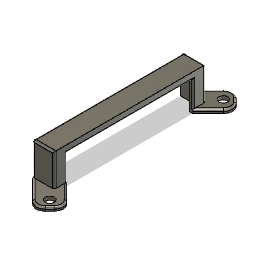
halterung_hdbaset_sender v1 (Autodesk Fusion 360 design; units mm, degrees)
Autodesk Fusion 360 part; units mm, degrees
note: some values were not read from the file. Chosen so that the rebuilt part matches the saved one: which pieces of a blend or face edit are solid.
sketch "Skizze1" plane through (0, 0, 0) normal (1, 0, 0) x (0, 0, -1)
  line L0 (0, 0) -> (0, 18)
  line L1 (0, 18) -> (80, 18)
  line L2 (80, 18) -> (80, 0)
  line L3 (0, 0) -> (-2, 0)
  line L4 (-2, 0) -> (-2, 20)
  line L5 (-2, 20) -> (82, 20)
  line L6 (82, 20) -> (82, 0)
  line L7 (82, 0) -> (80, 0)
  dimension "d1" = 18
  dimension "d2" = 80
  dimension "d3" = 18
  dimension "d4" = 2
  dimension "d5" = 20
  dimension "d6" = 84
  constraint coincident L0.start L3.start
  constraint vertical L0
  constraint perpendicular L0 L1
  constraint perpendicular L1 L2
  constraint perpendicular L0 L3
  constraint perpendicular L3 L4
  constraint perpendicular L4 L5
  constraint perpendicular L3 L6
  constraint perpendicular L2 L7
  measures "d1" distance of L0.start L0.end
  measures "d2" distance of L0.end L1.end
  measures "d3" distance of L1.end L2.end
  measures "d4" distance of L0.start L3.end
  measures "d5" distance of L3.end L4.end
  measures "d6" distance of L4.end L5.end
extrude "Extrusion1" add sketch "Skizze1" along normal blind 10
sketch "Skizze2" plane through (10, 0, 0) normal (1, 0, 0) x (0, 0, -1)
  line L0 (0, 0) -> (0, 18)
  line L1 (0, 18) -> (80, 18)
  line L2 (80, 18) -> (80, 0)
  line L3 (80, 0) -> (82, 0)
  line L4 (82, 0) -> (82, 20)
  line L5 (82, 20) -> (-2, 20)
  line L6 (-2, 20) -> (-2, 0)
  line L7 (-2, 0) -> (0, 0)
  line L8 (-2, 20) -> (-2, 0)
  line L9 (-2, 0) -> (5, 0)
  line L10 (5, 0) -> (5, 16)
  line L11 (5, 16) -> (75, 16)
  line L12 (75, 16) -> (75, 0)
  line L13 (75, 0) -> (82, 0)
  line L14 (82, 20) -> (82, 0)
  line L15 (82, 20) -> (-2, 20)
  dimension "d9" = 7
  dimension "d10" = 16
  dimension "d11" = 7
  constraint coincident L5.end L6.start
  constraint coincident L6.end L7.start
  constraint perpendicular L0 L9
  constraint perpendicular L9 L10
  constraint perpendicular L10 L11
  constraint perpendicular L1 L12
  constraint coincident L3.end L4.start
  constraint perpendicular L4 L13
  constraint coincident L4.end L5.start
  measures "d9" distance of L6.end L9.end
  measures "d10" distance of L9.end L10.end
  measures "d11" distance of L12.end L3.end
extrude "Extrusion2" add sketch "Skizze2" along normal blind 2
ref_plane "Arbeitsebene1" through (6, 0, -1.5) normal (0, -1, 0) x (0, 0, -1)
sketch "Skizze3" plane through (6, 0, -1.5) normal (0, -1, 0) x (1, 0, 0)
  line L0 (-6, 3.5) -> (4.949747, 14.449747)
  line L1 (12.020815, 14.449747) -> (14.449747, 12.020815)
  line L2 (14.449747, 4.949747) -> (6, -3.5)
  line L3 (6, -73.5) -> (14.449747, -81.949747)
  line L4 (14.449747, -89.020815) -> (12.020815, -91.449747)
  line L5 (4.949747, -91.449747) -> (-6, -80.5)
  line L6 (6, 3.5) -> (6, -3.5)
  line L7 (6, -73.5) -> (6, -80.5)
  circle A0 centre (9.722718, 9.676777) radius 2.5
  circle A1 centre (9.676777, -86.722718) radius 2.5
  arc A2 (12.020815, 14.449747) -> (4.949747, 14.449747) centre (8.485281, 10.914214) ccw
  arc A3 (14.449747, 4.949747) -> (14.449747, 12.020815) centre (10.914214, 8.485281) ccw
  arc A4 (14.449747, -89.020815) -> (14.449747, -81.949747) centre (10.914214, -85.485281) ccw
  arc A5 (4.949747, -91.449747) -> (12.020815, -91.449747) centre (8.485281, -87.914214) ccw
  line L8 (-6, -80.5) -> (6, -80.5)
  line L9 (6, -80.5) -> (6, -73.5)
  line L10 (-6, 3.5) -> (6, 3.5)
  line L11 (6, 3.5) -> (6, -3.5)
  point P0 (6, -73.5)
  point P1 (-6, -80.5)
  point P2 (6, -3.5)
  point P3 (-6, 3.5)
  dimension "d15" = 45
  dimension "d16" = 45
  dimension "d17" = 12
  dimension "d18" = 12
  dimension "d19" = 5
  dimension "d20" = 6.75
  dimension "d21" = 5
  dimension "d22" = 6.75
  dimension "d23" = 5
  dimension "d24" = 5
  dimension "d25" = 5
  constraint perpendicular L0 L1
  constraint perpendicular L1 L2
  constraint perpendicular L3 L4
  constraint perpendicular L4 L5
  constraint coincident P0 L3.start
  constraint coincident P1 L5.end
  constraint coincident L2.end L6.end
  constraint coincident P3 L0.start
  constraint tangent L0 A2
  constraint tangent L1 A2
  constraint tangent L1 A3
  constraint tangent L2 A3
  constraint equal A2 A3
  constraint tangent L3 A4
  constraint tangent L4 A4
  constraint equal A2 A4
  constraint tangent L4 A5
  constraint tangent L5 A5
  constraint equal A2 A5
  constraint coincident L7.end L8.end
  constraint coincident L6.start L10.end
  measures "d15" angle of L2 L6
  measures "d16" angle of L3 L7
  measures "d17" distance of L4 L7.end
  measures "d18" distance of L1 L6.start
  measures "d19" diameter of A0
  measures "d21" diameter of A1
  measures "d25" radius of A2
extrude "Extrusion3" add sketch "Skizze3" against normal blind 2
fillet "Abrundung1" radius 1 20 edges at (6, 20, 2) (6, 20, -82) (12, 11, -82) (12, 9, -75) (12, 16, -40) (16.224874, 2, -79.224874) (21.914214, 2, -86.985281) (19.235281, 2, -91.735281) (14.485281, 2, -94.414214) (5.474874, 2, -87.474874) (12, 9, -5) (12, 11, 2) (0, 11, 2) (5.474874, 2, 7.474874) (14.485281, 2, 14.414214) (19.235281, 2, 11.735281) (21.914214, 2, 6.985281) (16.224874, 2, -0.775126) (0, 20, -40) (0, 11, -82)
